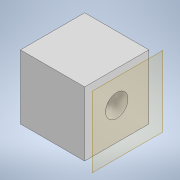
# Autodesk Inventor part: test_part_01
Saved by Autodesk Inventor 2020 (Build 240168000, 168)
## iProperties
Created: 2019-11-09
Part Number: test_part_01
Material: Generic
Document SubType Name: Modeling
Designer: maste
Density: 1 g/cm^3
Appearance: Default
Author: maste
Autodesk Inventor part; units mm, degrees
ref_plane "YZ Plane" through (0, 0, 0) normal (1, 0, 0) x (0, 1, 0)
ref_plane "XZ Plane" through (0, 0, 0) normal (0, 1, 0) x (-1, 0, 0)
ref_plane "XY Plane" through (0, 0, 0) normal (0, 0, 1) x (1, 0, 0)
sketch "Sketch1" plane through (0, 0, 0) normal (1, 0, 0) x (0, 1, 0)
  line L0 (0, 0) -> (12, 0)
  line L1 (12, 0) -> (12, -12)
  line L2 (12, -12) -> (0, -12)
  line L3 (0, -12) -> (0, 0)
  dimension "d0" = 12
  dimension "d1" = 12
  constraints: 8 end point, 2 parallel, 1 horizontal, 1 perpendicular
  measures "d0" distance of L1.end L2.end
  measures "d1" distance of L0.end L1.end
extrude "Extrusion1" add sketch "Sketch1" along normal blind 12
ref_plane "Work Plane1" through (14, 0, 0) normal (1, 0, 0) x (0, 0, -1)
sketch "Sketch2" plane through (14, 0, 0) normal (1, 0, 0) x (0, 0, -1)
  arc A0 (6, 3.1) -> (6, 8.9) centre (6, 6) ccw
  line L0 (6, 6) -> (6, 8.9)
  line L1 (6, 6) -> (6, 3.1)
  point P0 (0, 0)
  dimension "d5" = 5.8
  dimension "d6" = 6
  dimension "d7" = 6
  constraints: 4 end point, 2 point on circle, 1 centre point, 1 point on line, 1 vertical
  measures "d5" diameter of A0
  measures "d6" horizontal distance of point (0, 0) L0.start
  measures "d7" horizontal distance of point (0, 0) L0.start
revolve "Revolution1" cut sketch "Sketch2" angle 360 about axis through (14, 6, -6) along (0, 1, 0)
body "Solid1"
